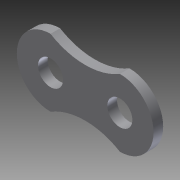
# Autodesk Inventor part: inner_link
Saved by Autodesk Inventor 2011 SP1 (Build 150282100, 282)
## iProperties
Created: 2013-01-14
Part Number: inner_link
Document SubType Name: Modeling
Designer: 971065
Density: 1 g/cm^3
Author: 971065
Autodesk Inventor part; units mm, degrees
ref_plane "YZ Plane" through (0, 0, 0) normal (1, 0, 0) x (0, 1, 0)
ref_plane "XZ Plane" through (0, 0, 0) normal (0, 1, 0) x (-1, 0, 0)
ref_plane "XY Plane" through (0, 0, 0) normal (0, 0, 1) x (1, 0, 0)
sketch "Sketch1" plane through (0, 0, 0) normal (0, 0, 1) x (1, 0, 0)
  line L0 (-30.8649, 3.175) -> (-30.8649, -3.175)
  circle A0 centre (-35.4369, 0) radius 1.651
  circle A1 centre (-26.2929, 0) radius 1.651
  arc A2 (-35.4369, 4.445) -> (-26.2929, 4.445) centre (-30.8649, 12.0396) ccw
  arc A3 (-26.2929, -4.445) -> (-35.4369, -4.445) centre (-30.8649, -12.0396) ccw
  arc A4 (-26.2929, -4.445) -> (-26.2929, 4.445) centre (-26.2929, 0) ccw
  arc A5 (-35.4369, 4.445) -> (-35.4369, -4.445) centre (-35.4369, 0) ccw
  point P0 (0, 0)
  dimension "d2" = 6.35
  dimension "d3" = 3.175
  dimension "d4" = 3.175
  dimension "d6" = 4.572
  dimension "d7" = 9.144
  dimension "d8" = 3.302
  dimension "d9" = 3.302
  constraints: 10 point on circle, 6 centre point, 2 coincident, 2 end point, 1 vertical
  measures "d2" distance of L0.start L0.end
  measures "d3" vertical distance of A4.centre L0.start
  measures "d4" vertical distance of L0.end A5.centre
  measures "d6" distance from line of A5.centre L0
  measures "d7" distance of A4.centre A5.centre
  measures "d8" diameter of A0
  measures "d9" diameter of A1
extrude "Extrusion1" add sketch "Sketch1" along normal blind 1.27
body "Solid1"
